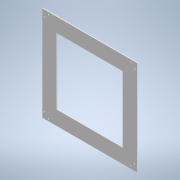
# Autodesk Inventor part: Hinterwand
Saved by Autodesk Inventor 2021 (Build 250183000, 183)
## iProperties
Created: 2022-06-27
Part Number: Hinterwand
Material: Generisch
Document SubType Name: Modeling
Designer: adria
Mass: 608.831 g
Surface Area: 2614.99 cm^2
Volume: 608.831 cm^3
Density: 1 g/cm^3
Appearance: Vorgabe
Author: adria
Autodesk Inventor part; units mm, degrees
ref_plane "YZ Plane" through (0, 0, 0) normal (1, 0, 0) x (0, 1, 0)
ref_plane "XZ Plane" through (0, 0, 0) normal (0, 1, 0) x (-1, 0, 0)
ref_plane "XY Plane" through (0, 0, 0) normal (0, 0, 1) x (1, 0, 0)
sketch "Skizze1" plane through (0, 0, 0) normal (0, 0, 1) x (1, 0, 0)
  line L0 (-250, -250) -> (250, -250)
  line L1 (250, -250) -> (250, 250)
  line L2 (250, 250) -> (-250, 250)
  line L3 (-250, 250) -> (-250, -250)
  line L4 (-250, -250) -> (250, 250) construction
  line L5 (250, -250) -> (-250, 250) construction
  point P0 (0, 0)
  dimension "d0" = 500
  dimension "d1" = 500
  constraints: 12 end point, 2 midpoint, 2 parallel, 1 horizontal, 1 perpendicular
  measures "d0" distance of L2.end L1.end
  measures "d1" distance of L1.end L0.end
extrude "Extrusion1" add sketch "Skizze1" along normal blind 5
sketch "Skizze2" plane through (0, 0, 5) normal (0, 0, 1) x (1, 0, 0)
  line L0 (250, 250) -> (-250, 250) projected
  line L1 (-250, 250) -> (-250, -250) projected
  line L2 (0, -350) -> (0, 350) projected
  line L3 (-350, 0) -> (350, 0) projected
  point P0 (0, 0)
  point P1 (-238, 217)
  point P2 (-217, 238)
  point P3 (238, 217)
  point P4 (217, 238)
  point P5 (-238, -217)
  point P6 (-217, -238)
  point P7 (217, -238)
  point P8 (238, -217)
  dimension "d4" = 33
  dimension "d5" = 33
  dimension "d6" = 12
  dimension "d7" = 12
  constraints: 6 symmetric about line
  measures "d4" distance from line of L0 point (-238, 217)
  measures "d5" distance from line of L1 point (-217, 238)
  measures "d6" distance from line of L0 point (-217, 238)
  measures "d7" distance from line of L1 point (-238, 217)
hole "Bohrung1" at (-238, 217, 5) at (-217, 238, 5) at (217, 238, 5) at (238, 217, 5) at (-238, -217, 5) at (-217, -238, 5) at (217, -238, 5) at (238, -217, 5) direction (0, 0, -1) diameter 6.1 end through all
sketch "Skizze3" plane through (0, 0, 5) normal (0, 0, 1) x (1, 0, 0)
  line L0 (-160, -200) -> (160, -200)
  line L1 (160, -200) -> (160, 200)
  line L2 (160, 200) -> (-160, 200)
  line L3 (-160, 200) -> (-160, -200)
  line L4 (-160, -200) -> (160, 200) construction
  line L5 (160, -200) -> (-160, 200) construction
  point P0 (0, 0)
  dimension "d15" = 320
  dimension "d16" = 400
  constraints: 12 end point, 2 midpoint, 2 parallel, 1 horizontal, 1 perpendicular
  measures "d15" distance of L2.end L1.end
  measures "d16" distance of L1.end L0.end
extrude "Extrusion2" cut sketch "Skizze3" against normal through all
